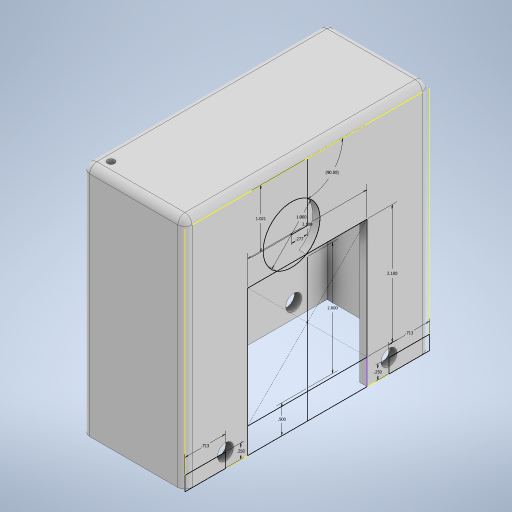
# Autodesk Inventor part: ThermalOvershield
Saved by Autodesk Inventor 2024.1 (Build 281209000, 209)
## iProperties
Created: 2024-08-21
Part Number: ThermalOvershield
Material: Generic
Document SubType Name: Modeling
Designer: pab2
Density: 1 g/cm^3
Appearance: Default
Author: pab2
Autodesk Inventor part; units mm, degrees
ref_plane "YZ Plane" through (0, 0, 0) normal (1, 0, 0) x (0, 1, 0)
ref_plane "XZ Plane" through (0, 0, 0) normal (0, 1, 0) x (-1, 0, 0)
ref_plane "XY Plane" through (0, 0, 0) normal (0, 0, 1) x (1, 0, 0)
sketch "Sketch1" plane through (0, 0, 0) normal (0, 1, 0) x (-1, 0, 0)
  line L0 (0, 0) -> (25.4, 0)
  line L1 (25.4, 0) -> (25.4, -101.6)
  line L2 (25.4, -101.6) -> (0, -101.6)
  line L3 (0, -101.6) -> (0, 0)
  line L4 (25.4, 0) -> (31.75, 0)
  line L5 (31.75, 0) -> (31.75, -101.6)
  line L6 (31.75, -101.6) -> (25.4, -101.6)
  line L7 (25.4, -101.6) -> (25.4, 0)
  line L8 (0, -101.6) -> (-6.35, -101.6)
  line L9 (-6.35, -101.6) -> (-6.35, 0)
  line L10 (-6.35, 0) -> (0, 0)
  line L11 (0, 0) -> (0, -101.6)
  line L12 (-6.985, 0.635) -> (32.385, 0.635)
  line L13 (32.385, 0.635) -> (32.385, -102.235)
  line L14 (32.385, -102.235) -> (-6.985, -102.235)
  line L15 (-6.985, -102.235) -> (-6.985, 0.635)
  line L16 (-6.985, 0.635) -> (32.385, -102.235) construction
  line L17 (32.385, 0.635) -> (-6.985, -102.235) construction
  line L18 (-10.16, 3.81) -> (35.56, 3.81)
  line L19 (35.56, 3.81) -> (35.56, -105.41)
  line L20 (35.56, -105.41) -> (-10.16, -105.41)
  line L21 (-10.16, -105.41) -> (-10.16, 3.81)
  line L22 (-10.16, 3.81) -> (35.56, -105.41) construction
  line L23 (35.56, 3.81) -> (-10.16, -105.41) construction
  point P0 (12.7, -50.8)
  dimension "d0" = 25.4
  dimension "d1" = 101.6
  dimension "d2" = 6.35
  dimension "d3" = 6.35
  dimension "d4" = 39.37
  dimension "d5" = 102.87
  dimension "d6" = 45.72
  dimension "d7" = 109.22
  constraints: 48 end point, 10 parallel, 5 horizontal, 5 perpendicular, 4 midpoint, 1 point on line
  measures "d0" distance of L1.end L2.end
  measures "d1" distance of L0.end L1.end
  measures "d2" distance of L5.end L6.end
  measures "d3" distance of L9.end L10.end
  measures "d4" distance of L13.end L14.end
  measures "d5" distance of L12.end L13.end
  measures "d6" distance of L19.end L20.end
  measures "d7" distance of L18.end L19.end
extrude "Extrusion1" add sketch "Sketch1" along normal blind 101.6 contours L18 L19 L20 L21
sketch "Sketch2" plane through (10.16, 0, 3.81) normal (1, 0, 0) x (0, 0, -1)
  line L0 (109.22, 0) -> (109.22, 101.6) projected
  line L1 (109.22, 0) -> (91.1225, 0)
  line L2 (91.1225, 0) -> (91.1225, 6.35)
  line L3 (91.1225, 6.35) -> (109.22, 6.35)
  line L4 (109.22, 6.35) -> (109.22, 0)
  line L5 (106.045, 0) -> (3.175, 0) projected
  line L6 (54.61, 0) -> (54.61, 12.7)
  line L7 (54.61, 12.7) -> (54.61, 63.5)
  line L8 (27.94, 11.43) -> (81.28, 11.43)
  line L9 (81.28, 11.43) -> (81.28, 64.77)
  line L10 (81.28, 64.77) -> (27.94, 64.77)
  line L11 (27.94, 64.77) -> (27.94, 11.43)
  line L12 (27.94, 11.43) -> (81.28, 64.77) construction
  line L13 (81.28, 11.43) -> (27.94, 64.77) construction
  line L14 (27.94, 11.43) -> (81.28, 11.43)
  line L15 (81.28, 11.43) -> (81.28, 0)
  line L16 (81.28, 0) -> (27.94, 0)
  line L17 (27.94, 0) -> (27.94, 11.43)
  line L18 (106.045, 101.6) -> (3.175, 101.6) projected
  line L19 (54.61, 101.6) -> (54.61, 75.6666)
  line L20 (54.61, 101.6) -> (80.5434, 101.6) construction
  line L21 (54.61, 75.6666) -> (47.5742, 75.6666)
  circle A0 centre (47.5742, 75.6666) radius 12.7
  line L22 (0, 0) -> (0, 101.6) projected
  line L23 (0, 0) -> (18.0975, 0)
  line L24 (18.0975, 0) -> (18.0975, 6.35)
  line L25 (18.0975, 6.35) -> (0, 6.35)
  line L26 (0, 6.35) -> (0, 0)
  point P0 (3.81, 0)
  point P1 (25.4, 6.35)
  point P2 (54.61, 38.1)
  point P3 (41.0508, 64.77)
  point P4 (54.0976, 64.77)
  dimension "d12" = 18.0975
  dimension "d13" = 6.35
  dimension "d14" = 12.7
  dimension "d15" = 50.8
  dimension "d16" = 53.34
  dimension "d17" = 53.34
  dimension "d30" = 25.9334
  dimension "d31" = 90
  dimension "d37" = 7.0358
  dimension "d38" = 25.4
  dimension "d48" = 18.0975
  dimension "d49" = 6.35
  constraints: 46 end point, 8 parallel, 6 horizontal, 5 midpoint, 5 perpendicular, 2 point on line, 2 vertical, 1 centre point, 1 coincident
  measures "d12" distance of L2.end L3.end
  measures "d13" distance of L1.end L2.end
  measures "d14" distance of L6.start L6.end
  measures "d15" distance of L6.end L7.end
  measures "d16" distance of L10.end L9.end
  measures "d17" distance of L9.end L8.end
  measures "d30" distance of L19.start L19.end
  measures "d31" angle of L19 L20
  measures "d37" distance of L19.end L21.end
  measures "d38" diameter of A0
  measures "d48" distance of L25.end L24.end
  measures "d49" distance of L24.end L23.end
extrude "Extrusion2" cut sketch "Sketch2" against normal blind 3.175 contours L5 L6 L8 L15 | L5 L17 L8 L6 | L8 L11 L10 A0 L9 | A0 L10 picked at (46.2278, 64.3887)
hole "Hole1" at (10.16, 6.35, -87.3125) at (10.16, 6.35, -14.2875) direction (-1, 0, 0) diameter 7.1374 end through all clearance for "Socket Head Cap Screw" size "1/4" standard "Ansi Unified Screw Threads"
sketch "Sketch3" plane through (0, 101.6, 0) normal (0, 1, 0) x (1, 0, 0)
  line L0 (10.16, -3.81) -> (10.16, 105.41) projected
  line L1 (-35.56, -3.81) -> (10.16, -3.81)
  line L2 (10.16, -3.81) -> (10.16, 105.41)
  line L3 (10.16, 105.41) -> (-35.56, 105.41)
  line L4 (-35.56, 105.41) -> (-35.56, -3.81)
  point P0 (0, 0)
  constraints: 8 end point, 2 parallel, 1 horizontal, 1 perpendicular
extrude "Extrusion3" add sketch "Sketch3" along normal blind 3.175
fillet "Fillet1" radius 3.175 8 edges at (-12.7, 104.775, 3.81) (10.16, 52.3875, 3.81) (10.16, 104.775, -50.8) (-12.7, 104.775, -105.41) (10.16, 52.3875, -105.41) (-35.56, 104.775, -50.8) (-35.56, 52.3875, 3.81) (-35.56, 52.3875, -105.41)
extrude "Extrusion4" cut sketch "Sketch2" against normal through all contours L10 A0 picked at (51.5957, 75.6184)
sketch "Sketch4" plane through (0, 104.775, 0) normal (0, 1, 0) x (1, 0, 0)
  line L0 (-32.3579, -0.635) -> (-29.1829, -0.635)
  line L1 (-29.1829, -0.635) -> (-29.1829, 2.54)
  line L2 (-29.1829, 2.54) -> (-32.3579, 2.54)
  line L3 (-32.3579, 2.54) -> (-32.3579, -0.635)
  point P0 (0, 0)
  dimension "d39" = 3.175
  dimension "d40" = 3.175
  constraints: 8 end point, 2 parallel, 1 horizontal, 1 perpendicular
  measures "d39" distance of L2.end L1.end
  measures "d40" distance of L1.end L0.end
hole "Hole2" at (-29.1829, 104.775, -2.54) direction (0, -1, 0) diameter 3.175 end through all
body "Solid1"
